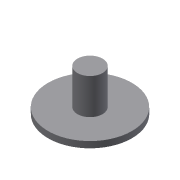
# Autodesk Inventor part: CYLINDER
Saved by Autodesk Inventor 2022 Beta2 (Build 260130000, 130) ContinuousBuild 0
## iProperties
Created: 2013-05-20
Part Number: CYLINDER
Material: Generic
Document SubType Name: Modeling
Designer: czachry
Density: 1 g/cm^3
Appearance: Default
Author: czachry
Autodesk Inventor part; units mm, degrees
ref_plane "YZ Plane" through (0, 0, 0) normal (1, 0, 0) x (0, 1, 0)
ref_plane "XZ Plane" through (0, 0, 0) normal (0, 1, 0) x (-1, 0, 0)
ref_plane "XY Plane" through (0, 0, 0) normal (0, 0, 1) x (1, 0, 0)
sketch "Sketch4" plane through (0, 0, 0) normal (0, 1, 0) x (-1, 0, 0)
  line L0 (0, 0) -> (0, 13.7009) construction
  line L1 (0, 0) -> (20, 0)
  line L2 (20, 0) -> (20, 3)
  line L3 (20, 3) -> (6, 3)
  line L4 (6, 3) -> (6, 20)
  line L5 (6, 20) -> (0, 20)
  line L6 (0, 20) -> (0, 0)
  dimension "d1" = 20
  dimension "d2" = 6
  dimension "d3" = 20
  dimension "d4" = 3
  constraints: 14 end point, 4 perpendicular, 2 parallel, 1 point on line, 1 vertical
  measures "d1" distance between parallel lines of L1 L5
  measures "d2" distance between parallel lines of L0 L4
  measures "d3" distance between parallel lines of L0 L2
  measures "d4" distance between parallel lines of L1 L3
revolve "Revolution1" add sketch "Sketch4" angle 360 about axis through (0, 0, 0) along (0, 0, 1)
body "Solid1"
